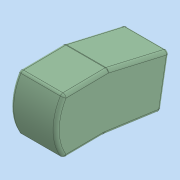
# Autodesk Inventor part: Wrist2
Saved by Autodesk Inventor 2020.2 (Build 242310000, 310)
## iProperties
Created: 2020-02-07
Part Number: Wrist2
Material: Aluminium 6061
Document SubType Name: Modeling
Designer: JochenAlt
Density: 2.7 g/cm^3
Appearance: Aluminium - dunkel
Author: JochenAlt
Autodesk Inventor part; units mm, degrees
ref_plane "YZ Plane" through (0, 0, 0) normal (1, 0, 0) x (0, 1, 0)
ref_plane "XZ Plane" through (0, 0, 0) normal (0, 1, 0) x (-1, 0, 0)
ref_plane "XY Plane" through (0, 0, 0) normal (0, 0, 1) x (1, 0, 0)
sketch "Main" plane through (0, 0, 0) normal (1, 0, 0) x (0, 1, 0)
  line L0 (-46.9756, 0) -> (44.6362, 0) construction
  arc A0 (-12.0367, -4.9109) -> (-12.6859, -2.8403) centre (0, 0) ccw
  arc A1 (26.5, 40.3851) -> (-26.5, 40.3851) centre (0, 0) ccw
  circle A2 centre (-6.54, 40.6533) radius 1.1
  circle A3 centre (-6.54, 40.6533) radius 2
  circle A4 centre (-9.8219, 22.0404) radius 1.1
  circle A5 centre (-9.8219, 22.0404) radius 2
  circle A6 centre (-14.5104, -4.5494) radius 2
  circle A7 centre (-14.5104, -4.5494) radius 1.1
  circle A8 centre (20.0498, 35.9648) radius 1.1
  circle A9 centre (20.0498, 35.9648) radius 2
  circle A10 centre (16.7679, 17.3519) radius 1.1
  circle A11 centre (16.7679, 17.3519) radius 2
  circle A12 centre (12.0794, -9.2379) radius 1.1
  circle A13 centre (12.0794, -9.2379) radius 2
  arc A14 (-12.0484, -4.9835) -> (-12.6859, -2.8403) centre (-14.5104, -4.5494) ccw
  line L1 (-14.1953, 20.273) -> (-10.2561, 19.5784)
  line L2 (-14.0763, -2.0874) -> (-18.0156, -1.3928)
  line L3 (20.273, 14.1953) -> (16.3337, 14.8899)
  line L4 (14.3058, 17.786) -> (18.4003, 41.0068)
  line L5 (16.4527, -7.4705) -> (20.273, 14.1953)
  line L6 (-7.3599, 21.6063) -> (-3.2655, 44.8271)
  line L7 (-14.1953, 20.273) -> (-18.0156, -1.3928)
  line L8 (10.5536, -61.0816) -> (-30.8083, -53.7884)
  line L9 (-14.9187, -10.8959) -> (-22.7329, -55.2123) construction
  line L10 (-11.508, -43.3817) -> (-29.2345, -40.2561) construction
  line L11 (-29.2345, -40.2561) -> (-29.0262, -39.0743) construction
  line L12 (-29.0262, -39.0743) -> (-11.2996, -42.2) construction
  line L13 (-11.508, -43.3817) -> (-11.2996, -42.2) construction
  line L14 (-2.1897, -44.0094) -> (-12.9944, -42.1042) construction
  line L15 (-12.9944, -42.1042) -> (-13.5154, -45.0586) construction
  line L16 (-13.5154, -45.0586) -> (-2.7106, -46.9638) construction
  line L17 (-2.7106, -46.9638) -> (-2.1897, -44.0094) construction
  line L18 (-12.9944, -42.1042) -> (-27.4008, -39.564) construction
  line L19 (-27.4008, -39.564) -> (-27.9217, -42.5184) construction
  line L20 (-27.9217, -42.5184) -> (-13.5154, -45.0586) construction
  line L21 (5.8901, -58.7361) -> (4.9053, -58.5625)
  line L22 (-24.8945, -49.0432) -> (-23.9097, -49.2168)
  line L23 (6.6194, -54.5999) -> (5.8901, -58.7361)
  line L24 (4.9053, -58.5625) -> (4.6448, -60.0397) construction
  line L25 (5.6346, -54.4263) -> (5.895, -52.9491)
  line L26 (5.895, -52.9491) -> (6.8799, -53.1227)
  line L27 (6.6194, -54.5999) -> (5.6346, -54.4263)
  line L28 (-24.634, -47.566) -> (-23.6492, -47.7396)
  line L29 (-23.6492, -47.7396) -> (-23.9097, -49.2168)
  line L30 (-23.9097, -49.2168) -> (6.6194, -54.5999) construction
  line L31 (6.8799, -53.1227) -> (7.6092, -48.9865)
  line L32 (7.6092, -48.9865) -> (11.253, -49.629)
  line L33 (-23.9047, -43.4298) -> (-27.5485, -42.7873)
  line L34 (7.6092, -48.9865) -> (-8.1477, -46.2082)
  line L35 (-8.1477, -46.2082) -> (-23.9047, -43.4298)
  line L36 (-8.1477, -46.2082) -> (-10.1273, -57.435)
  line L37 (4.9053, -58.5625) -> (-24.639, -53.353) construction
  line L38 (4.9053, -58.5625) -> (4.6448, -60.0397)
  line L39 (-24.639, -53.353) -> (-24.8995, -54.8303)
  line L40 (-24.639, -53.353) -> (-25.6238, -53.1794)
  line L41 (6.6194, -54.5999) -> (11.5434, -55.4682)
  line L42 (-24.8945, -49.0432) -> (-29.8185, -48.175)
  line L43 (-24.634, -47.566) -> (-23.9047, -43.4298)
  line L44 (13.3826, -61.5804) -> (27.0531, -2.3668)
  line L45 (-30.8083, -53.7884) -> (-28.7773, -42.2698)
  line L46 (-24.6683, -9.1768) -> (-29.9819, -39.3119)
  line L47 (12.5847, -49.563) -> (10.5536, -61.0816)
  line L48 (14.7283, -47.1956) -> (20.042, -17.0604)
  arc A15 (-29.9819, -39.3119) -> (-27.5485, -42.7873) centre (-27.0275, -39.8329) ccw
  arc A16 (11.253, -49.629) -> (14.7283, -47.1956) centre (11.7739, -46.6746) ccw
  line L49 (0, -83.5571) -> (0, 70.28) construction
  line L50 (7.5674, 42.9169) -> (0, 0) construction
  line L51 (20.273, 14.1953) -> (24.2806, 36.9237)
  line L52 (-10.1877, 43.0014) -> (-14.1953, 20.273)
  line L53 (21.8471, 40.399) -> (-6.7123, 45.4348)
  line L54 (16.4527, -7.4705) -> (12.5135, -6.7759)
  arc A17 (12.5135, -6.7759) -> (9.6173, -8.8038) centre (12.0794, -9.2379) ccw
  line L55 (9.6173, -8.8038) -> (8.6065, -14.5364)
  line L56 (20.0498, 35.9648) -> (12.0794, -9.2379) construction
  arc A18 (14.3058, 17.786) -> (16.3337, 14.8899) centre (16.7679, 17.3519) ccw
  line L57 (-6.54, 40.6533) -> (20.0498, 35.9648) construction
  line L58 (-6.54, 40.6533) -> (-14.5104, -4.5494) construction
  arc A19 (-10.2561, 19.5784) -> (-7.3599, 21.6063) centre (-9.8219, 22.0404) ccw
  line L59 (16.7679, 17.3519) -> (-9.8219, 22.0404) construction
  line L60 (12.0794, -9.2379) -> (-14.5104, -4.5494) construction
  arc A20 (-18.4186, -3.6785) -> (-13.0556, -10.6955) centre (-12.5097, -4.7204) ccw
  line L61 (-18.0156, -1.3928) -> (-18.4186, -3.6785)
  line L62 (-24.6683, -9.1768) -> (-14.9187, -10.8959)
  line L63 (-13.0556, -10.6955) -> (-12.0484, -4.9835)
  line L64 (-23.9047, -43.4298) -> (-24.634, -47.566)
  line L65 (-8.1477, -46.2082) -> (-2.3132, -13.1186) construction
  line L66 (-25.6238, -53.1794) -> (-24.8945, -49.0432)
  line L67 (-24.634, -47.566) -> (-23.9047, -43.4298)
  line L68 (-14.9187, -10.8959) -> (8.5197, -15.0288)
  line L69 (8.6102, -14.5158) -> (8.5197, -15.0288)
  line L70 (8.5197, -15.0288) -> (20.042, -17.0604)
  line L71 (26.5, 40.3851) -> (27.0531, -2.3668)
  line L72 (14.7283, -47.1956) -> (16.6263, -47.5302) construction
  line L73 (-12.0484, -4.9835) -> (-13.1461, -11.2085)
  line L74 (16.4527, -7.4705) -> (16.0497, -9.7562)
  arc A21 (8.6102, -14.5158) -> (16.0497, -9.7562) centre (10.1408, -8.7143) ccw
  line L75 (-18.4186, -3.6785) -> (-19.5473, -10.0798)
  line L76 (16.0497, -9.7562) -> (14.921, -16.1575)
  arc A22 (-6.7123, 45.4348) -> (-10.1877, 43.0014) centre (-7.2332, 42.4804) ccw
  arc A23 (24.2806, 36.9237) -> (21.8471, 40.399) centre (21.3262, 37.4446) ccw
  line L77 (8.6065, -14.5364) -> (-13.5516, -10.6293) construction
  line L78 (-14.8526, -2.5789) -> (-12.8084, -2.2239)
  line L79 (-13.6663, -6.3625) -> (-11.7854, -5.4868)
  arc A24 (-12.6859, -2.8403) -> (-12.0367, -4.9109) centre (0, 0) ccw
  arc A25 (-12.6859, -2.8403) -> (-14.0763, -2.0874) centre (-14.5104, -4.5494) ccw
  line L80 (13.0748, -7.5032) -> (11.2753, -6.4705)
  line L81 (10.666, -10.653) -> (9.198, -9.1868)
  line L82 (-26.0843, 2.2821) -> (-33.8882, -53.2453)
  line L83 (-26.5, 40.3851) -> (-26.0843, 2.2821)
  line L84 (27.0531, -2.3668) -> (-26.0843, 2.2821) construction
  line L85 (20.042, -17.0604) -> (23.5193, -17.6736)
  line L86 (-24.6683, -9.1768) -> (-27.6216, -8.6561)
  line L87 (-29.1137, -34.3879) -> (15.5966, -42.2715)
  line L88 (-10.1273, -57.435) -> (-10.301, -58.4198)
  line L89 (10.5536, -61.0816) -> (13.3826, -61.5804)
  line L90 (-30.8083, -53.7884) -> (-33.8882, -53.2453)
  line L91 (-31.9068, -39.1471) -> (-29.9983, -39.4154) construction
  line L92 (-10.301, -58.4198) -> (0, -60.2361) construction
  line L93 (6.8799, -53.1227) -> (11.8039, -53.991)
  line L94 (-24.634, -47.566) -> (-29.558, -46.6977)
  line L95 (5.895, -52.9491) -> (-23.6492, -47.7396)
  line L96 (22.8109, 40.0515) -> (23.9053, 41.9731) construction
  line L97 (24.3259, 37.4834) -> (26.5372, 37.512) construction
  point P0 (31.5488, 36.577)
  point P1 (9.2125, -14.3622)
  point P2 (10.473, -14.5845)
  point P3 (8.6102, -14.5158)
  point P4 (-13.0556, -10.6955)
  point P5 (-13.3747, -2.3223)
  point P6 (0, 48.3032)
  dimension "d86" = 26
  dimension "d188" = 27
  dimension "d189" = 18.9
  dimension "d190" = 5
  dimension "d393" = 35
  dimension "d400" = 4
  dimension "d401" = 2.2
  dimension "d443" = 18
  dimension "d445" = 3
  dimension "d446" = 14.6286
  dimension "d447" = 10.9714
  dimension "d448" = 0.2
  dimension "d449" = 32
  dimension "d450" = 4.2
  dimension "d451" = 1.5
  dimension "d452" = 1
  dimension "d453" = 1.5
  dimension "d458" = 0.2
  dimension "d459" = 58.321
  dimension "d474" = 3
  dimension "d476" = 45.4
  dimension "d481" = 42
  dimension "d482" = 22
  dimension "d487" = 7
  dimension "d489" = 6
  dimension "d491" = 9.9
  dimension "d499" = 31.4
  dimension "d503" = 1.9273
  dimension "d530" = 3
  dimension "d533" = 27
  dimension "d535" = 56.4
  dimension "d541" = 12.821
  dimension "d542" = 10
  dimension "d543" = 95
  dimension "d544" = 3
  dimension "d545" = 2
  dimension "d546" = 0.5
  dimension "d561" = 8
  dimension "d586" = 58.4198
  dimension "d587" = 1
  dimension "d589" = 48
  dimension "d590" = 53
  dimension "d593" = 45
  dimension "d613" = 10.4599
  dimension "d226" = 32
  dimension "d322" = 0.2
  dimension "d324" = 38
  dimension "d336" = 1
  dimension "d337" = 0.2
  dimension "d519" = 1
  dimension "d553" = 30
  dimension "d554" = 2.2
  dimension "d555" = 4
  dimension "d563" = 18
  dimension "d564" = 39
  dimension "d565" = 6.7
  dimension "d566" = 2.5
  dimension "d568" = 2
  dimension "d208" = 20
  dimension "d210" = 1
  dimension "d241" = 5
  dimension "d247" = 13
  dimension "d263" = 2.2
  dimension "d264" = 2
  dimension "d265" = 3
  dimension "d266" = 0.2
  dimension "d307" = 4.5
  dimension "d381" = 0.2
  dimension "d594" = 0.1
  dimension "d306" = 4.5
  constraints: 192 end point, 48 point on circle, 44 perpendicular, 29 point on line, 26 centre point, 26 collinear, 25 tangent, 14 equal radius, 13 coincident, 9 parallel, 8 line through centre, 3 equal length, 2 midpoint, 11 other
  measures "d86" diameter of A0
  measures "d188" distance of A5.centre A6.centre
  measures "d189" distance of A2.centre A4.centre
  measures "d190" diameter of A14
  measures "d393" distance between parallel lines of L7 L5
  measures "d400" diameter of A3
  measures "d401" diameter of A2
  measures "d443" distance of L10.start L10.end
  measures "d445" distance of L16.end L14.start
  measures "d446" distance of L19.end L15.end
  measures "d447" distance of L15.end L16.end
  measures "d448" distance between parallel lines of L18 L12
  measures "d449" distance of L21.start L40.end
  measures "d450" distance of L23.start L21.start
  measures "d451" distance between parallel lines of L8 L21
  measures "d452" distance of L21.end L21.start
  measures "d453" distance of L25.start L25.end
  measures "d458" distance between parallel lines of L16 L34
  measures "d459" distance from line of A0.centre L8
  measures "d474" radius of A15
  measures "d476" distance between parallel lines of L46 L48
  measures "d481" distance of L8.start L8.end
  measures "d482" distance between parallel lines of L6 L4
  measures "d487" distance from line of L60 L50.end
  measures "d489" radius of A20
  measures "d491" distance between parallel lines of L46 L9
  measures "d499" distance between parallel lines of L10 L62
  measures "d503" distance of L48.start L72.end
  measures "d530" radius of A22
  measures "d533" distance between parallel lines of L58 L56
  measures "d535" distance between parallel lines of L77 L53
  measures "d541" distance from line of L77 L50.end
  measures "d542" angle of L49 L65
  measures "d543" angle of L65 L84
  measures "d544" angle of L44 L48
  measures "d545" angle of L46 L82
  measures "d546" distance of L68.end L55.end
  measures "d561" distance between parallel lines of L87 L34
  measures "d586" vertical distance of L88.end L50.end
  measures "d587" distance of L36.end L88.end
  measures "d589" distance of L82.end L44.start
  measures "d590" distance of L83.start L71.start
  measures "d593" distance between parallel lines of L8 L68
  measures "d613" distance of L88.end L92.end
extrude "BodyStart" add sketch "Main" along normal mid plane 44 contours A14 A0 A17 | A0 L79 L63 A14 | A24 A14 | A14 L63 L79 A6 L78 A25 A24 | A0 L81 L55 L69 L68 L73 L63 L79 | A25 L78 A0 | A0 A17 L55 L81 | L63 A20 L61 L2 A25 L78 A6 L79 | L78 A25 L2 L7 L1 A19 L6 L53 L4 A18 L3 L5 L54 A17 L80 A0 | A17 A0 | A0 A17 L80 A13 L81 L55 | L81 A13 L80 A17 L54 L74 A21 L55 | L73 L68 L62 L75 A20 | A6 | L80 A17 A0 | A21 L76 L70 L69 L55 | A13 | L75 L62 L86 L82 L83 A1 L71 L44 L85 L70 L76 L74 L5 L51 A23 L53 A22 L52 L7 L61 | L68 L70 L48 L87 L46 L62 | L52 A22 L53 L6 A19 L1 | L46 A15 L45 L90 L82 L86 | L3 A18 L4 L53 A23 L51 | L85 L44 L89 L47 A16 L48 | L87 L48 A16 L32 L34 L35 L33 A15 L46 | A15 L33 L43 L94 L45 | L45 L42 L66 L40 L39 L8 | L47 L93 L31 L32 A16 | L8 L38 L21 L23 L41 L47 | L94 L28 L29 L22 L42 L45 | L39 L40 L66 L22 L29 L95 L36 L8 | L47 L41 L27 L25 L26 L93 | L8 L36 L95 L25 L27 L23 L21 L38 | L43 L35 L36 L95 L28 | L26 L95 L36 L34 L31 | A2 | A3 | A4 | A5 | A7 | A8 | A9 | A10 | A11 | A12
fillet "Rundung18" radius 3 18 edges at (-22, 26.7766, 19.0091) (-22, 20.2178, -31.9736) (0, 13.3826, -61.5804) (-22, -10.2528, -57.4128) (0, -33.8882, -53.2453) (22, 20.2178, -31.9736) (22, -10.2528, -57.4128) (0, 27.0531, -2.3668) (22, 26.7766, 19.0091) (0, 26.5, 40.3851) (-22, 0, 48.3032) (-22, -26.2922, 21.3336) (-22, -29.9863, -25.4816) (0, -26.0843, 2.2821) (0, -26.5, 40.3851) (22, 0, 48.3032) (22, -26.2922, 21.3336) (22, -29.9863, -25.4816)
sketch "Skizze9" plane through (-31, 0, 0) normal (-1, 0, 0) x (0, 0, 1)
  circle A0 centre (-5.15, 0) radius 1.1 projected
  circle A1 centre (5.15, 0) radius 1.1 projected
  arc A2 (-6.3066, 1.6316) -> (-6.3066, -1.6316) centre (-5.15, 0) ccw
  arc A3 (6.3066, -1.6316) -> (6.3066, 1.6316) centre (5.15, 0) ccw
  arc A4 (2.5, 4.3301) -> (-2.5, 4.3301) centre (0, 0) ccw construction
  arc A5 (-2.5, -4.3301) -> (2.5, -4.3301) centre (0, 0) ccw construction
  line L0 (-6.3066, -1.6316) -> (-2.5, -4.3301)
  line L1 (-6.3066, 1.6316) -> (-2.5, 4.3301)
  line L2 (2.5, 4.3301) -> (6.3066, 1.6316)
  line L3 (6.3066, -1.6316) -> (2.5, -4.3301)
  line L4 (-2.5, 4.3301) -> (-2.5, -4.3301)
  line L5 (2.5, 4.3301) -> (2.5, -4.3301)
  point P0 (0, 0)
  dimension "d299" = 4
  dimension "d620" = 5
  dimension "d599" = 2
  dimension "d600" = 2
  dimension "d601" = 2
  dimension "d602" = 2
  dimension "d603" = 1
  dimension "d604" = 2
  dimension "d605" = 2
  dimension "d606" = 2
  dimension "d607" = 0.2
  dimension "d608" = 0.2
  dimension "d621" = 2
  dimension "d622" = 2
  dimension "d623" = 1
  dimension "d625" = 1
  constraints: 32 end point, 20 point on circle, 13 tangent, 10 centre point, 6 parallel, 1 coincident, 21 other
  measures "d602" distance between parallel lines of L3 L4
  measures "d605" distance between parallel lines of L2 L5
  measures "d621" radial gap between concentric circles of A2 A3
equation "\"roundness_small\" = 3"
equation "\"roundness_tiny\" = 0.5"
equation "\"wall_thickness\" = 3"
equation "\"medium_arm_width\" = 51"
equation "\"big_arm_width\" = 56"
equation "\"bevel_angle\" = 20deg"
equation "\"medium_arm_radius\" = 35"
equation "\"big_arm_radius\" = 48"
equation "\"medium_arm_circle_centre\" = 11"
equation "\"big_arm_circle_centre\" = 25"
equation "\"thickness\" = 3"
equation "\"press_fit\" = 0.1"
equation "\"tight_fit\" = 0.2"
equation "\"m2_hex_width\" = 4.2"
equation "\"m2_washer_diameter\" = 5.2"
equation "\"m2_screw_hole_diameter\" = 2.2"
equation "\"m2_allen_screw_width\" = 4"
equation "\"m2_allen_screw_height\" = 2"
equation "\"m2_washer_height\" = 0.3"
